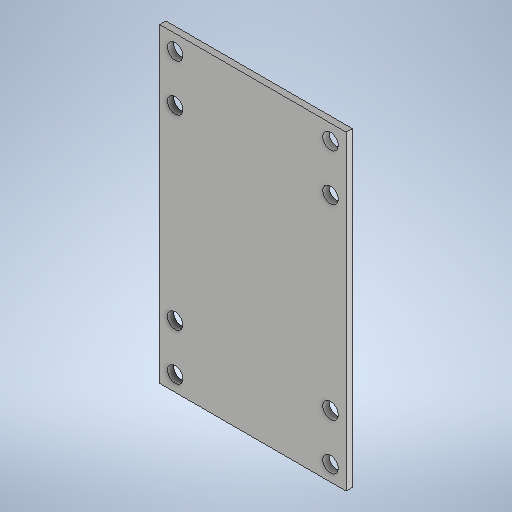
# Autodesk Inventor part: Сrane plate 1
Saved by Autodesk Inventor 2025 (Build 290162010, 162A)
## iProperties
Created: 2024-06-15
Part Number: Сrane plate 1
Material: Generic
Document SubType Name: Sheet Metal
Designer: admin
Density: 1 g/cm^3
Sheet Metal Rule: Default
Appearance: Default
Stock Number: Кран Пластина 1
Flat Pattern Width: 24 cm
Flat Pattern Length: 40 cm
Flat Pattern Area: 960 cm^2
Sheet Metal Width: 240,000 mm
Sheet Metal Length: 400,000 mm
Sheet Metal Area: 96000,000 mm^2
Author: admin
Autodesk Inventor part; units mm, degrees
ref_plane "YZ Plane" through (0, 0, 0) normal (1, 0, 0) x (0, 1, 0)
ref_plane "XZ Plane" through (0, 0, 0) normal (0, 1, 0) x (-1, 0, 0)
ref_plane "XY Plane" through (0, 0, 0) normal (0, 0, 1) x (1, 0, 0)
sketch "Sketch1" plane through (0, 0, 0) normal (0, 1, 0) x (-1, 0, 0)
  line L0 (120, -200) -> (-120, -200)
  line L1 (-120, -200) -> (-120, 200)
  line L2 (-120, 200) -> (120, 200)
  line L3 (120, 200) -> (120, -200)
  line L4 (120, -200) -> (-120, 200) construction
  line L5 (-120, -200) -> (120, 200) construction
  point P0 (0, 0)
  point P1 (0, 0)
  dimension "d16" = 240
  dimension "d17" = 400
  measures "d16" distance of L1.end L2.end
  measures "d17" distance of L0.end L1.end
extrude "Plate1" add sketch "Sketch1" along normal blind 8
sketch "Sketch2" plane through (0, 0, 0) normal (0, -1, 0) x (1, 0, 0)
  line L0 (100, 180) -> (100, -180) construction
  line L1 (-120, -200) -> (120, -200) projected
  line L2 (120, -200) -> (120, 200) projected
  line L3 (120, 200) -> (-120, 200) projected
  line L4 (-120, 200) -> (-120, -200) projected
  point P0 (100, 0)
  point P1 (100, 0)
  point P2 (0, 0)
  point P3 (100, 120)
  point P4 (100, -120)
  dimension "d19" = 20
  dimension "d20" = 20
  dimension "d21" = 360
  dimension "d22" = 120
  dimension "d23" = 120
  constraints: 2 coincident, 2 end point, 2 point on line, 1 horizontal alignment, 1 midpoint, 1 vertical
  measures "d19" distance between parallel lines of L2 L0
  measures "d20" distance from line of L0.start L3
  measures "d21" distance of L0.start L0.end
  measures "d22" distance of point (100, 0) point (100, -120)
  measures "d23" distance of point (100, 0) point (100, 120)
hole "Hole1" at (100, 0, 180) at (100, 0, -180) at (100, 0, -120) at (100, 0, 120) direction (0, 1, 0) diameter 20 end through all
mirror "Mirror1" about plane through (0, 0, 0) normal (1, 0, 0) of "Hole1"
equation "\"d20\" = d19"
equation "\"d23\" = d22"
equation "\"d3\" = d19"
equation "\"d8\" = Thickness"
equation "\"d2\" = Thickness"
equation "\"BendRadius\" = Thickness"
equation "\"BendReliefWidth\" = Thickness"
equation "\"BendReliefDepth\" = 0.5 * Thickness"
equation "\"CornerReliefSize\" = 4 * Thickness"
equation "\"MinimumRemnant\" = 2 * Thickness"
equation "\"TransitionRadius\" = BendRadius"
equation "\"JacobiRadiusSize\" = BendRadius"
equation "\"GapSize\" = Thickness"
equation "\"Thickness\" = 8"
body "Solid1"
